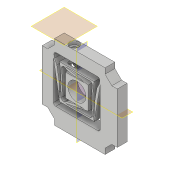
# Autodesk Inventor part: 50_Cube_Insert_Thorlabs
Saved by Autodesk Inventor 2019.4 (Build 234330000, 330)
## iProperties
Created: 2019-07-01
Part Number: 50_Cube_Insert_Thorlabs
Material: Generic
Document SubType Name: Modeling
Designer: diederichbenedict
Density: 1 g/cm^3
Appearance: Default
Author: diederichbenedict
Autodesk Inventor part; units mm, degrees
ref_plane "YZ Plane" through (0, 0, 0) normal (1, 0, 0) x (0, 1, 0)
ref_plane "Work Plane1" through (0, 0, 10) normal (0, 0, 1) x (1, 0, 0)
sketch "Sketch1" plane through (0, 0, 10) normal (0, 0, 1) x (1, 0, 0)
  line L0 (-4.0299, -0.3538) -> (-2.2322, 1.4439) construction
  arc A0 (-1.4439, 2.2322) -> (-2.2322, 1.4439) centre (-0.9299, 0.9299) ccw construction
  line L1 (-1.4439, 2.2322) -> (0.3538, 4.0299) construction
  line L2 (-37.8299, 42.2137) -> (-37.8299, 45.8299) construction
  line L3 (-37.8299, 45.8299) -> (-4.0299, 45.8299) construction
  line L4 (-4.0299, 45.8299) -> (-4.0299, 42.2137) construction
  line L5 (-4.0299, 4.0299) -> (0.3538, 4.0299) projected
  line L6 (-20.9299, 58.9723) -> (17.1124, 20.9299) construction
  line L7 (17.1124, 20.9299) -> (-20.9299, -17.1124) construction
  line L8 (-20.9299, -17.1124) -> (-58.9723, 20.9299) construction
  line L9 (-58.9723, 20.9299) -> (-20.9299, 58.9723) construction
  line L10 (-20.9299, 58.9723) -> (-20.9299, -17.1124) construction
  line L11 (17.1124, 20.9299) -> (-58.9723, 20.9299) construction
  line L12 (-20.9299, 58.9723) -> (32.8701, 58.9723) construction
  line L13 (-43.4299, 43.4299) -> (1.5701, 43.4299) construction
  line L14 (1.5701, 43.4299) -> (1.5701, -1.5701) construction
  line L15 (1.5701, -1.5701) -> (-43.4299, -1.5701) construction
  line L16 (-43.4299, -1.5701) -> (-43.4299, 43.4299) construction
  line L17 (-43.4299, 43.4299) -> (1.5701, -1.5701) construction
  line L18 (1.5701, 43.4299) -> (-43.4299, -1.5701) construction
  line L19 (-43.4299, 5.3876) -> (-43.4299, 36.4723)
  line L20 (-43.4299, 36.4723) -> (-36.4723, 43.4299)
  line L21 (-36.4723, 43.4299) -> (-5.3876, 43.4299)
  line L22 (-5.3876, 43.4299) -> (1.5701, 36.4723)
  line L23 (1.5701, 36.4723) -> (1.5701, 5.3876)
  line L24 (1.5701, 5.3876) -> (-5.3876, -1.5701)
  line L25 (-5.3876, -1.5701) -> (-36.4723, -1.5701)
  line L26 (-36.4723, -1.5701) -> (-43.4299, 5.3876)
  line L27 (-4.0299, 42.2137) -> (-37.8299, 42.2137) projected
  line L28 (-4.0299, -0.3538) -> (-4.0299, 4.0299) projected
  circle A1 centre (-20.9299, 20.9299) radius 13.3985
  circle A2 centre (-20.9299, 20.9299) radius 15.4895
  point P0 (-37.8299, 4.0299)
  dimension "d18" = 53.8
  dimension "d19" = 45
  dimension "d20" = 53.8
  dimension "d21" = 45
  dimension "d22" = 45
  dimension "d30" = 26.797
  dimension "d36" = 30.979
  constraints: 42 end point, 15 point on line, 4 parallel, 3 midpoint, 3 perpendicular, 2 centre point, 2 coincident, 2 horizontal, 1 equal length
  measures "d18" distance of L6.start L6.end
  measures "d19" angle of L6 L12
  measures "d20" distance of L6.end L7.end
  measures "d21" distance of L14.end L15.end
  measures "d22" distance of L13.end L14.end
  measures "d30" diameter of A1
  measures "d36" diameter of A2
extrude "Extrusion1" add sketch "Sketch1" along normal blind 6.5 contours L28 L24 L25 L26 L19 L20 L27 L22 L23 L5 | L5 L24 L28 | L27 L20 L21 L22 | A1 | A2
ref_plane "Work Plane2" through (-40.9959, 0.8639, 22.2359) normal (0, 0, 1) x (1, 0, 0)
sketch "Sketch3" plane through (0, 0, 10) normal (0, 0, -1) x (-1, 0, 0)
  line L0 (37.8299, -0.4701) -> (37.8299, 4.0299) construction
  line L1 (4.0299, 4.0299) -> (4.0299, -0.4701) construction
  line L2 (37.8299, -0.4701) -> (37.8299, 1.1886) construction
  line L3 (4.0299, -3.9701) -> (4.0299, -0.3538) construction
  line L4 (45.8299, 4.0299) -> (42.2137, 4.0299) construction
  line L5 (-0.3538, 4.0299) -> (-3.9701, 4.0299) construction
  line L6 (-3.9701, 37.8299) -> (-0.3538, 37.8299) construction
  line L7 (4.0299, 42.2137) -> (4.0299, 45.8299) construction
  line L8 (37.8299, 45.8299) -> (37.8299, 42.2137) construction
  line L9 (42.2137, 37.8299) -> (45.8299, 37.8299) construction
  line L10 (37.8299, 37.7299) -> (45.8299, 37.7299)
  line L11 (45.8299, 37.7299) -> (45.8299, 4.1299)
  line L12 (45.8299, 4.1299) -> (37.8299, 4.1299)
  line L13 (37.8299, 4.1299) -> (37.8299, 37.7299)
  line L14 (37.7299, 4.0299) -> (4.1299, 4.0299)
  line L15 (4.1299, 4.0299) -> (4.1299, -3.9701)
  line L16 (4.1299, -3.9701) -> (37.7299, -3.9701)
  line L17 (37.7299, -3.9701) -> (37.7299, 4.0299)
  line L18 (4.0299, 4.1299) -> (-3.9701, 4.1299)
  line L19 (-3.9701, 4.1299) -> (-3.9701, 37.7299)
  line L20 (-3.9701, 37.7299) -> (4.0299, 37.7299)
  line L21 (4.0299, 37.7299) -> (4.0299, 4.1299)
  line L22 (4.1299, 37.8299) -> (37.7299, 37.8299)
  line L23 (37.7299, 37.8299) -> (37.7299, 45.8299)
  line L24 (37.7299, 45.8299) -> (4.1299, 45.8299)
  line L25 (4.1299, 45.8299) -> (4.1299, 37.8299)
  point P0 (0, 0)
  dimension "d23" = 0.1
  dimension "d24" = 0.1
  dimension "d25" = 0.1
  dimension "d26" = 0.1
  dimension "d27" = 0.1
  constraints: 32 end point, 8 parallel, 4 horizontal, 4 perpendicular, 3 point on line
  measures "d23" distance between parallel lines of L8 L23
  measures "d24" distance between parallel lines of L7 L25
  measures "d25" distance between parallel lines of L6 L20
  measures "d26" distance between parallel lines of L5 L18
  measures "d27" distance between parallel lines of L1 L15
extrude "Extrusion3" add sketch "Sketch3" against normal up to surface (6.5 mm away)
sketch "Sketch11" plane through (0, 0, 16.5) normal (0, 0, 1) x (1, 0, 0)
  line L0 (3.9701, 4.1299) -> (0.3124, 4.1299) projected
  line L1 (3.9701, 37.7299) -> (3.9701, 4.1299) projected
  line L2 (0.3124, 37.7299) -> (3.9701, 37.7299) projected
  line L3 (0.3124, 37.7299) -> (-4.1299, 42.1723) projected
  line L4 (-4.1299, 45.8299) -> (-4.1299, 42.1723) projected
  line L5 (-37.7299, 45.8299) -> (-4.1299, 45.8299) projected
  line L6 (-37.7299, 42.1723) -> (-37.7299, 45.8299) projected
  line L7 (-37.7299, 42.1723) -> (-42.1723, 37.7299) projected
  line L8 (-45.8299, 37.7299) -> (-42.1723, 37.7299) projected
  line L9 (-45.8299, 4.1299) -> (-45.8299, 37.7299) projected
  line L10 (-42.1723, 4.1299) -> (-45.8299, 4.1299) projected
  line L11 (-42.1723, 4.1299) -> (-37.7299, -0.3124) projected
  line L12 (-37.7299, -3.9701) -> (-37.7299, -0.3124) projected
  line L13 (-4.1299, -3.9701) -> (-37.7299, -3.9701) projected
  line L14 (-4.1299, -0.3124) -> (-4.1299, -3.9701) projected
  line L15 (-4.1299, -0.3124) -> (0.3124, 4.1299) projected
  circle A0 centre (-22.8299, 22.8299) radius 6
  point P0 (0, 0)
  dimension "d0" = 12
  dimension "d88" = 23
  dimension "d89" = 23
  constraints: 1 centre point
  measures "d0" diameter of A0
  measures "d88" distance from line of A0.centre L5
  measures "d89" distance from line of L9 A0.centre
extrude "Extrusion7" cut sketch "Sketch11" against normal through all contours A0
sketch "Sketch12" plane through (0, 0, 16.5) normal (0, 0, 1) x (1, 0, 0)
  circle A0 centre (-22.8299, 22.8299) radius 6 projected
  line L0 (3.9701, 4.1299) -> (0.3124, 4.1299) projected
  line L1 (3.9701, 37.7299) -> (3.9701, 4.1299) projected
  line L2 (0.3124, 37.7299) -> (3.9701, 37.7299) projected
  line L3 (0.3124, 37.7299) -> (-4.1299, 42.1723) projected
  line L4 (-4.1299, 45.8299) -> (-4.1299, 42.1723) projected
  line L5 (-37.7299, 45.8299) -> (-4.1299, 45.8299) projected
  line L6 (-37.7299, 42.1723) -> (-37.7299, 45.8299) projected
  line L7 (-37.7299, 42.1723) -> (-42.1723, 37.7299) projected
  line L8 (-45.8299, 37.7299) -> (-42.1723, 37.7299) projected
  line L9 (-45.8299, 4.1299) -> (-45.8299, 37.7299) projected
  line L10 (-42.1723, 4.1299) -> (-45.8299, 4.1299) projected
  line L11 (-42.1723, 4.1299) -> (-37.7299, -0.3124) projected
  line L12 (-37.7299, -3.9701) -> (-37.7299, -0.3124) projected
  line L13 (-4.1299, -3.9701) -> (-37.7299, -3.9701) projected
  line L14 (-4.1299, -0.3124) -> (-4.1299, -3.9701) projected
  line L15 (-4.1299, -0.3124) -> (0.3124, 4.1299) projected
  line L16 (-15.3299, 15.3299) -> (-30.3299, 15.3299)
  line L17 (-30.3299, 15.3299) -> (-30.3299, 30.3299)
  line L18 (-30.3299, 30.3299) -> (-15.3299, 30.3299)
  line L19 (-15.3299, 30.3299) -> (-15.3299, 15.3299)
  line L20 (-15.3299, 15.3299) -> (-30.3299, 30.3299) construction
  line L21 (-30.3299, 15.3299) -> (-15.3299, 30.3299) construction
  line L22 (-7.3299, 38.3299) -> (-38.3299, 38.3299)
  line L23 (-38.3299, 38.3299) -> (-38.3299, 7.3299)
  line L24 (-38.3299, 7.3299) -> (-7.3299, 7.3299)
  line L25 (-7.3299, 7.3299) -> (-7.3299, 38.3299)
  point P0 (0, 0)
  dimension "d1" = 15
  dimension "d93" = 15
  dimension "d94" = 8
  constraints: 20 end point, 4 parallel, 2 midpoint, 2 perpendicular, 1 horizontal, 3 other
  measures "d1" distance of L17.end L18.end
  measures "d93" distance of L16.end L17.end
  measures "d94" distance between parallel lines of L18 L22
extrude "Extrusion8" cut sketch "Sketch12" against normal through all contours L25 L24 L23 L22
sketch "Sketch13" plane through (0, 0, 16.5) normal (0, 0, 1) x (1, 0, 0)
  line L0 (-15.3299, 15.3299) -> (-15.3299, 30.3299) projected
  line L1 (-15.3299, 30.3299) -> (-30.3299, 30.3299) projected
  line L2 (-30.3299, 30.3299) -> (-30.3299, 15.3299) projected
  line L3 (-30.3299, 15.3299) -> (-15.3299, 15.3299) projected
  circle A0 centre (-22.8299, 22.8299) radius 6 projected
  line L4 (3.9701, 4.1299) -> (0.3124, 4.1299) projected
  line L5 (3.9701, 37.7299) -> (3.9701, 4.1299) projected
  line L6 (0.3124, 37.7299) -> (3.9701, 37.7299) projected
  line L7 (0.3124, 37.7299) -> (-4.1299, 42.1723) projected
  line L8 (-4.1299, 45.8299) -> (-4.1299, 42.1723) projected
  line L9 (-37.7299, 45.8299) -> (-4.1299, 45.8299) projected
  line L10 (-37.7299, 42.1723) -> (-37.7299, 45.8299) projected
  line L11 (-37.7299, 42.1723) -> (-42.1723, 37.7299) projected
  line L12 (-45.8299, 37.7299) -> (-42.1723, 37.7299) projected
  line L13 (-45.8299, 4.1299) -> (-45.8299, 37.7299) projected
  line L14 (-42.1723, 4.1299) -> (-45.8299, 4.1299) projected
  line L15 (-42.1723, 4.1299) -> (-37.7299, -0.3124) projected
  line L16 (-37.7299, -3.9701) -> (-37.7299, -0.3124) projected
  line L17 (-4.1299, -3.9701) -> (-37.7299, -3.9701) projected
  line L18 (-4.1299, -0.3124) -> (-4.1299, -3.9701) projected
  line L19 (-4.1299, -0.3124) -> (0.3124, 4.1299) projected
  line L20 (-38.3299, 7.3299) -> (-38.3299, 38.3299) projected
  line L21 (-38.3299, 38.3299) -> (-7.3299, 38.3299) projected
  line L22 (-7.3299, 38.3299) -> (-7.3299, 7.3299) projected
  line L23 (-7.3299, 7.3299) -> (-38.3299, 7.3299) projected
  line L24 (-30.3299, 15.3299) -> (-15.3299, 15.3299) projected
  line L25 (-30.3299, 30.3299) -> (-15.3299, 30.3299) projected
  line L26 (-15.3299, 30.3299) -> (-19.3299, 30.3299)
  line L27 (-38.3299, 38.3299) -> (-7.3299, 38.3299) projected
  line L28 (-38.3299, 7.3299) -> (-38.3299, 38.3299) projected
  line L29 (-12.3289, 33.3309) -> (-33.333, 33.3309)
  line L30 (-33.3289, 12.3309) -> (-12.3289, 12.3309)
  line L31 (-12.3289, 33.3309) -> (-33.3289, 12.3309) construction
  line L32 (-33.333, 33.3309) -> (-12.3289, 12.3309) construction
  line L33 (-34.3265, 34.281) -> (-11.3789, 34.281)
  line L34 (-11.3789, 11.3809) -> (-34.322, 11.3809)
  line L35 (-33.333, 33.3309) -> (-18.3793, 30.3299)
  line L36 (-15.3299, 30.3299) -> (-30.2836, 33.3309)
  line L37 (-21.0064, 30.8572) -> (-24.564, 30.8572)
  line L38 (-24.564, 30.8572) -> (-29.6214, 31.8721)
  line L39 (-32.434, 32.4368) -> (-33.333, 33.3309)
  line L40 (-28.8299, 22.8299) -> (-16.8299, 22.8299)
  line L41 (-15.3299, 15.3299) -> (-15.3299, 30.3299) projected
  line L42 (-15.3299, 15.3299) -> (-30.2786, 12.3309)
  line L43 (-33.3289, 12.3309) -> (-18.3803, 15.3299)
  line L44 (-32.434, 13.2244) -> (-24.564, 14.8033)
  line L45 (-24.564, 14.8033) -> (-20.9542, 14.8136)
  line L46 (-30.2786, 12.3309) -> (-33.3289, 12.3309)
  line L47 (-29.622, 13.7886) -> (-30.5782, 12.8828)
  line L48 (-29.6214, 31.8721) -> (-30.5775, 32.778)
  arc A1 (-34.322, 11.3809) -> (-34.3265, 34.281) centre (-99.9562, 22.8181) ccw
  arc A2 (-33.3289, 12.3309) -> (-33.333, 33.3309) centre (-99.9562, 22.8181) ccw
  line L49 (-34.322, 11.3809) -> (-34.322, 12.3309)
  line L50 (-34.3265, 12.8448) -> (-34.3265, 34.281)
  line L51 (-33.333, 33.3309) -> (-33.333, 32.617)
  arc A3 (-11.3789, 34.281) -> (-11.3789, 11.3809) centre (57.145, 22.8309) ccw
  arc A4 (-12.3289, 33.3309) -> (-12.3289, 12.3309) centre (57.145, 22.8309) ccw
  line L52 (-12.3289, 28.4017) -> (-12.3289, 29.1157)
  line L53 (-12.3289, 29.7277) -> (-12.3289, 30.3299)
  line L54 (-12.3289, 30.8572) -> (-12.3289, 33.3309)
  line L55 (-11.3789, 34.281) -> (-11.3789, 16.1226)
  line L56 (-11.3789, 15.3299) -> (-11.3789, 11.3809)
  point P0 (0, 0)
  point P1 (-38.3299, 37.8299)
  point P2 (-40.3299, 39.5723)
  point P3 (-39.5723, 40.3299)
  dimension "d134" = 21
  dimension "d135" = 21
  dimension "d137" = 0.6
  dimension "d142" = 0.7
  dimension "d143" = 0.7
  dimension "d144" = 0
  dimension "d145" = 0
  dimension "d3" = 0.6
  constraints: 56 end point, 21 point on line, 13 parallel, 10 point on circle, 4 centre point, 4 horizontal, 4 tangent, 3 perpendicular, 2 concentric, 1 collinear, 3 other
  measures "d134" distance of L30.end L30.start
  measures "d135" distance of L30.start L29.end
  measures "d137" distance between parallel lines of L36 L35
  measures "d142" distance between parallel lines of L35 L38
  measures "d143" distance between parallel lines of L43 L44
  measures "d144" horizontal distance of L39.start L44.start
  measures "d145" horizontal distance of L37.end L44.end
  measures "d3" distance between parallel lines of L43 L42
extrude "Extrusion9" add sketch "Sketch13" against normal up to surface (6.5 mm away) contours L3 L2 L1 L0 | L42 L30 L43 L3 | L1 L35 L29 L36 | L43 L47 L44 L45 | L37 L38 L48 L35 | L4 L19 L18 L17 L16 L15 L14 L13 L12 L11 L10 L9 L8 L7 L6 L5 | L33 A3 L34 A1
ref_plane "Work Plane3" through (-34.3265, 22.8309, 16.5) normal (0, 1, 0) x (1, 0, 0)
sketch "Sketch14" plane through (0, 0, 10) normal (0, 0, -1) x (-1, 0, 0)
  line L0 (30.2786, 12.3309) -> (12.3289, 12.3309) construction
  line L1 (12.3289, 33.3309) -> (30.2836, 33.3309) construction
  line L2 (30.2836, 33.3309) -> (15.3299, 30.3299) construction
  line L3 (15.3299, 30.3299) -> (15.3299, 15.3299) construction
  line L4 (11.3789, 11.3809) -> (34.322, 11.3809) construction
  line L5 (34.3265, 34.281) -> (11.3789, 34.281) construction
  circle A0 centre (22.8299, 22.8299) radius 6 construction
  line L6 (18.3803, 15.3299) -> (30.3299, 15.3299) construction
  line L7 (30.3299, 15.3299) -> (30.3299, 30.3299) construction
  line L8 (30.3299, 30.3299) -> (18.3793, 30.3299) construction
  line L9 (18.3793, 30.3299) -> (21.0064, 30.8572) construction
  line L10 (21.0064, 30.8572) -> (24.564, 30.8572) construction
  line L11 (24.564, 30.8572) -> (29.6214, 31.8721) construction
  line L12 (38.3299, 38.3299) -> (38.3299, 7.3299) projected
  line L13 (38.3299, 7.3299) -> (7.3299, 7.3299) construction
  line L14 (7.3299, 7.3299) -> (7.3299, 38.3299) construction
  line L15 (7.3299, 38.3299) -> (38.3299, 38.3299) construction
  line L16 (45.8299, 37.7299) -> (45.8299, 4.1299) projected
  line L17 (-3.9701, 4.1299) -> (-3.9701, 37.7299) construction
  line L18 (-0.3124, 4.1299) -> (-3.9701, 4.1299) construction
  line L19 (-0.3124, 4.1299) -> (4.1299, -0.3124) construction
  line L20 (4.1299, -0.3124) -> (4.1299, -3.9701) construction
  line L21 (4.1299, -3.9701) -> (37.7299, -3.9701) construction
  line L22 (37.7299, -3.9701) -> (37.7299, -0.3124) projected
  line L23 (37.7299, -0.3124) -> (42.1723, 4.1299) projected
  line L24 (45.8299, 4.1299) -> (42.1723, 4.1299) construction
  line L25 (34.322, 11.3809) -> (38.3299, 34.5212)
  line L26 (38.3299, 38.3299) -> (38.3299, 7.3299) projected
  line L27 (38.3299, 38.3299) -> (34.0065, 13.3683)
  line L28 (38.3299, 34.5212) -> (38.3299, 38.3299)
  line L29 (38.3299, 38.3299) -> (37.7299, 37.0609)
  line L30 (36.7309, 34.9575) -> (34.646, 22.9198)
  line L31 (34.646, 22.9198) -> (34.602, 16.8061)
  line L32 (42.1723, 37.7299) -> (45.8299, 37.7299) projected
  line L33 (42.1723, 37.7299) -> (37.7299, 42.1723) projected
  line L34 (37.7299, 42.1723) -> (37.7299, 45.8299) projected
  line L35 (37.7299, 45.8299) -> (4.1299, 45.8299) projected
  line L36 (4.1299, 45.8299) -> (4.1299, 42.1723) projected
  line L37 (4.1299, 42.1723) -> (-0.3124, 37.7299) projected
  line L38 (-3.9701, 37.7299) -> (-0.3124, 37.7299) projected
  line L39 (29.622, 13.7886) -> (24.564, 14.8033) projected
  line L40 (24.564, 14.8033) -> (20.9542, 14.8136) projected
  line L41 (20.9542, 14.8136) -> (18.3803, 15.3299) projected
  line L42 (15.3299, 15.3299) -> (30.2786, 12.3309) projected
  line L43 (33.3289, 12.3309) -> (30.5782, 12.8828) projected
  line L44 (30.5782, 12.8828) -> (29.622, 13.7886) projected
  line L45 (29.6214, 31.8721) -> (30.5775, 32.778) projected
  line L46 (30.5775, 32.778) -> (33.333, 33.3309) projected
  line L47 (37.6821, 34.5895) -> (36.1367, 31.5267)
  arc A1 (33.333, 33.3309) -> (33.3289, 12.3309) centre (99.9562, 22.8181) ccw projected
  arc A2 (34.3265, 34.281) -> (34.322, 11.3809) centre (99.9562, 22.8181) ccw projected
  arc A3 (11.3789, 11.3809) -> (11.3789, 34.281) centre (-57.145, 22.8309) ccw projected
  arc A4 (12.3289, 12.3309) -> (12.3289, 33.3309) centre (-57.145, 22.8309) ccw projected
  arc A5 (34.3265, 34.281) -> (34.322, 11.3809) centre (99.9562, 22.8181) ccw projected
  point P0 (0, 0)
  dimension "d138" = 0.65
  dimension "d141" = 1
  constraints: 14 end point, 6 point on line, 2 parallel, 1 point on circle
  measures "d138" distance between parallel lines of L25 L27
  measures "d141" distance between parallel lines of L27 L30
extrude "Extrusion10" add sketch "Sketch14" against normal up to surface (6.5 mm away)
ref_plane "Work Plane4" through (-22.8299, 15.3299, 16.5) normal (-1, 0, 0) x (0, 0, 1)
mirror "Mirror2" about plane through (-22.8299, 15.3299, 16.5) normal (-1, 0, 0) of "Extrusion10"
ref_plane "Work Plane5" through (-37.7299, 49.6299, 10) normal (0, 1, 0) x (1, 0, 0)
sketch "Sketch8" plane through (-37.7299, 49.6299, 10) normal (0, 1, 0) x (1, 0, 0)
  line L0 (33.6, 0) -> (0, 0) projected
  line L1 (0, -6.5) -> (0, 0) projected
  line L2 (0, -6.5) -> (33.6, -6.5) projected
  line L3 (33.6, -6.5) -> (33.6, 0) projected
  point P0 (9.9675, -3.3147)
hole "Hole1" at (-27.7624, 49.6299, 13.3147) direction (0, -1, 0) diameter 2.9 end up to surface counterbore diameter 6 counterbore depth 6
sketch "Sketch9" plane through (-45.8299, 4.1299, 10) normal (1, 0, 0) x (0, 0, -1)
  line L0 (-6.5, 33.6) -> (-6.5, 0) projected
  line L1 (0, 0) -> (-6.5, 0) projected
  line L2 (0, 0) -> (0, 33.6) projected
  line L3 (0, 18.7898) -> (-6.5, 18.7898) projected
  line L4 (0, 33.6) -> (-6.5, 33.6) projected
  point P0 (-3.25, 18.7898)
  point P1 (0, 19.6702)
  point P2 (-6.5, 19.6702)
  constraints: 2 other
hole "Hole2" at (-45.8299, 22.9198, 13.25) direction (1, 0, 0) diameter 2.9 depth 11.5 tip angle 179 counterbore diameter 6 counterbore depth 6
sketch "Sketch15" plane through (-34.3265, 34.281, 16.5) normal (0, 1, 0) x (1, 0, 0)
  circle A0 centre (6.5641, 3.1853) radius 1.45 projected
  line L0 (4.5641, 3.1853) -> (8.5641, 3.1853) construction
  line L1 (4.5641, 1.5353) -> (8.5641, 1.5353)
  line L2 (8.5641, 4.8353) -> (4.5641, 4.8353)
  arc A1 (4.5641, 4.8353) -> (4.5641, 1.5353) centre (4.5641, 3.1853) ccw
  arc A2 (8.5641, 1.5353) -> (8.5641, 4.8353) centre (8.5641, 3.1853) ccw
  point P0 (34.3265, 16.5)
  dimension "d147" = 2
  dimension "d148" = 3.3
  constraints: 8 end point, 4 point on circle, 4 tangent, 2 centre point, 1 horizontal, 1 midpoint, 1 parallel
  measures "d147" distance of A0.centre L0.end
  measures "d148" diameter of A2
extrude "Extrusion11" cut sketch "Sketch15" against normal up to surface (3.951 mm away) contours A0 | A1 L2 A2 L1
sketch "Sketch16" plane through (-38.3299, 7.3299, 16.5) normal (1, 0, 0) x (0, 0, -1)
  circle A0 centre (3.25, 15.5898) radius 1.45 projected
  circle A1 centre (3.25, 15.5898) radius 1.65
  point P0 (16.5, -7.3299)
  dimension "d151" = 3.3
  constraints: 1 centre point, 1 coincident
  measures "d151" diameter of A1
extrude "Extrusion12" cut sketch "Sketch16" along normal blind 3 contours A0 | A1
fillet "Fillet2" radius 1.5 8 edges at (-33.333, 33.3309, 13.25) (-33.3289, 12.3309, 13.25) (-12.3289, 12.3309, 13.25) (-12.3289, 33.3309, 13.25) (-38.3299, 38.3299, 13.25) (-38.3299, 7.3299, 13.25) (-7.3299, 7.3299, 13.25) (-7.3299, 38.3299, 13.25)
body "Solid1"
